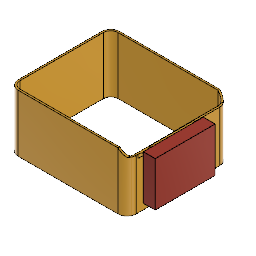
Assembly v4 (Autodesk Fusion 360 archive; units mm, degrees)
design "Battery Case 2"
Autodesk Fusion 360 part; units mm, degrees
sketch "Sketch1" plane through (0, 0, 0) normal (0, 0, 1) x (1, 0, 0) in component "Bottom"
  line L0 (78.75, -67.5) -> (-78.75, -67.5)
  line L1 (-78.75, -67.5) -> (-78.75, 67.5)
  line L2 (-78.75, 67.5) -> (78.75, 67.5)
  line L3 (78.75, 67.5) -> (78.75, -67.5)
  line L4 (78.75, -67.5) -> (-78.75, 67.5) construction
  line L5 (-78.75, -67.5) -> (78.75, 67.5) construction
  line L6 (81.25, -70) -> (-81.25, -70)
  line L7 (-81.25, -70) -> (-81.25, 70)
  line L8 (-81.25, 70) -> (81.25, 70)
  line L9 (81.25, 70) -> (81.25, -70)
  line L10 (81.25, -70) -> (-81.25, 70) construction
  line L11 (-81.25, -70) -> (81.25, 70) construction
  dimension "d1" = 157.5
  dimension "d2" = 135
  dimension "d4" = 2.5
  dimension "d5" = 2.5
  constraint horizontal L0
  constraint perpendicular L0 L1
  constraint parallel L0 L2
  constraint parallel L1 L3
  constraint coincident L4 origin
  constraint coincident L5 origin
  constraint horizontal L6
  constraint perpendicular L6 L7
  constraint parallel L6 L8
  constraint parallel L7 L9
  constraint coincident L10 origin
  constraint coincident L11 origin
  measures "d1" distance of L1.end L2.end
  measures "d2" distance of L0.end L1.end
  measures "d4" distance of L1 L7
  measures "d5" distance of L2 L8
extrude "Extrude2" add sketch "Sketch1" along normal blind 79 makes body 1 in component "Bottom"
fillet "Fillet4" radius 10 4 edges at (78.75, 67.5, 39.5) (-78.75, 67.5, 39.5) (-78.75, -67.5, 39.5) (78.75, -67.5, 39.5) on bodies 1 in component "Bottom"
fillet "Fillet4" radius 12.5 4 edges at (-81.25, -70, 39.5) (-81.25, 70, 39.5) (81.25, 70, 39.5) (81.25, -70, 39.5) on bodies 1 in component "Bottom"
sketch "Sketch4" plane through (0, 0, 79) normal (0, 0, 1) x (-1, 0, 0) in component "Bottom"
  arc A0 (-68.75, 70) -> (-81.25, 57.5) centre (-68.75, 57.5) ccw
  line L0 (-81.25, 57.5) -> (-81.25, -57.5)
  arc A1 (-81.25, -57.5) -> (-68.75, -70) centre (-68.75, -57.5) ccw
  line L1 (-68.75, -70) -> (68.75, -70)
  arc A2 (68.75, -70) -> (81.25, -57.5) centre (68.75, -57.5) ccw
  line L2 (81.25, -57.5) -> (81.25, 57.5)
  arc A3 (81.25, 57.5) -> (68.75, 70) centre (68.75, 57.5) ccw
  line L3 (68.75, 70) -> (-68.75, 70)
  line L4 (68.75, -67.5) -> (-68.75, -67.5)
  arc A4 (-78.75, -57.5) -> (-68.75, -67.5) centre (-68.75, -57.5) ccw
  line L5 (-78.75, -57.5) -> (-78.75, 57.5)
  arc A5 (-68.75, 67.5) -> (-78.75, 57.5) centre (-68.75, 57.5) ccw
  line L6 (-68.75, 67.5) -> (68.75, 67.5)
  arc A6 (78.75, 57.5) -> (68.75, 67.5) centre (68.75, 57.5) ccw
  line L7 (78.75, 57.5) -> (78.75, -57.5)
  arc A7 (68.75, -67.5) -> (78.75, -57.5) centre (68.75, -57.5) ccw
  line L8 (-68.75, -70) -> (-68.75, 70)
  constraint coincident A1.end L1.start
  constraint coincident A0.start L3.end
extrude "Extrude4" cut sketch "Sketch4" against normal up to surface (9 mm away) contours A0 L0 A1 A4 L5 A5 L8 bodies 1 in component "Bottom"
chamfer "Chamfer1" distance 9 angle 45 2 edges at (68.75, -68.75, 70) (68.75, 68.75, 70) on bodies 1 in component "Bottom"
sketch "Sketch5" plane through (81.25, 0, 0) normal (1, 0, 0) x (0, 1, 0) in component "Bottom"
  line L0 (57.5, 70) -> (-57.5, 70)
  line L1 (-57.5, 70) -> (-57.5, 0)
  line L2 (-57.5, 0) -> (57.5, 0)
  line L3 (57.5, 0) -> (57.5, 70)
  line L4 (15, 70) -> (15, 66)
  line L5 (15, 66) -> (-45, 66)
  line L6 (-45, 66) -> (-45, 70)
  dimension "d82" = 4
  dimension "d83" = 66
  dimension "d84" = 60
  dimension "d88" = 45
  constraint coincident L0 L4.start
  constraint perpendicular L0 L4
  constraint perpendicular L1 L5
  constraint coincident L0 L6.end
  constraint perpendicular L0 L6
  measures "d82" distance of L4.start L4.end
  measures "d83" distance of L2 L5
  measures "d84" distance of L4.end L5.end
  measures "d88" distance of origin L6
extrude "Extrude5" add sketch "Sketch5" along normal blind 6 contours L0 L4 L5 L6 bodies 1 in component "Bottom"
sketch "Sketch6" plane through (87.25, 0, 0) normal (1, 0, 0) x (0, 1, 0) in component "Bottom"
  line L0 (15, 70) -> (-45, 70)
  line L1 (-45, 66) -> (15, 66)
  line L2 (15, 66) -> (15, 70)
  line L3 (15, 70) -> (15, 78)
  line L4 (-45, 78) -> (-45, 70)
  line L5 (-45, 66) -> (-45, 48)
  line L6 (-45, 48) -> (15, 48)
  line L7 (15, 48) -> (15, 66)
  line L8 (-70, 79) -> (-67.5, 79)
  line L9 (-57.5, 79) -> (-67.5, 79)
  line L10 (-57.5, 79) -> (57.5, 79)
  line L11 (67.5, 79) -> (57.5, 79)
  line L12 (67.5, 79) -> (70, 79)
  line L13 (57.5, 79) -> (70, 79)
  line L14 (57.5, 79) -> (-57.5, 79)
  line L15 (-70, 79) -> (-57.5, 79)
  line L16 (-45, 70) -> (-45, 66)
  line L17 (-45, 78) -> (15, 78)
  dimension "d91" = 1
  dimension "d92" = 30
  constraint coincident L0.start L2.end
  constraint perpendicular L0 L3
  constraint coincident L0.end L4.end
  constraint coincident L1.start L5.start
  constraint perpendicular L1 L5
  constraint coincident L1.end L2.start
  constraint vertical L7
  constraint vertical L4
  constraint horizontal L17
  measures "d91" distance of L10 L17
  measures "d92" distance of L6 L17
extrude "Extrude6" add sketch "Sketch6" along normal blind 2.5 bodies 1 in component "Bottom"
chamfer "Chamfer2" distance 1 angle 45 3 edges at (87.25, -15, 66) (81.25, -15, 66) (87.25, -15, 70) on bodies 1 in component "Bottom"
fillet "Fillet5" radius 10 2 edges at (81.25, -45, 67.5) (81.25, 15, 67.5) on bodies 1 in component "Bottom"
sketch "Sketch1 (2)" plane through (0, 0, 0) normal (0, 0, 1) x (1, 0, 0) in component "BMS"
  line L0 (41.25, 30.75) -> (-41.25, 30.75)
  line L1 (-41.25, 30.75) -> (-41.25, -30.75)
  line L2 (-41.25, -30.75) -> (41.25, -30.75)
  line L3 (41.25, -30.75) -> (41.25, 30.75)
  line L4 (41.25, 30.75) -> (-41.25, -30.75) construction
  line L5 (-41.25, 30.75) -> (41.25, -30.75) construction
  dimension "d96" = 82.5
  dimension "d97" = 61.5
  constraint horizontal L0
  constraint perpendicular L0 L1
  constraint parallel L0 L2
  constraint parallel L1 L3
  constraint coincident L4 origin
  constraint coincident L5 origin
  measures "d96" distance of L1.end L2.end
  measures "d97" distance of L0.end L1.end
extrude "Extrude1" add sketch "Sketch1 (2)" along normal blind 16.5 separate body makes body 2 in component "BMS"
component "Bottom" placed x (1, 0, 0) y (0, 1, 0) z (0, 0, 1) at (0, 0, 0)
component "BMS" placed x (0, -1, 0) y (0, 0, 1) z (-1, 0, 0) at (106.25, -15, 47.25)
